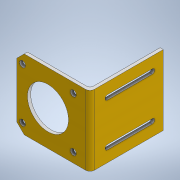
# Autodesk Inventor part: Soporte Motor
Saved by Autodesk Inventor 2021 (Build 250183000, 183)
## iProperties
Created: 2022-01-28
Part Number: Soporte Motor
Material: Generic
Document SubType Name: Modeling
Designer: deuts
Density: 1 g/cm^3
Appearance: Default
Author: deuts
Autodesk Inventor part; units mm, degrees
ref_plane "YZ Plane" through (0, 0, 0) normal (1, 0, 0) x (0, 1, 0)
ref_plane "XZ Plane" through (0, 0, 0) normal (0, 1, 0) x (-1, 0, 0)
ref_plane "XY Plane" through (0, 0, 0) normal (0, 0, 1) x (1, 0, 0)
sketch "Sketch1" plane through (0, 0, 0) normal (0, 1, 0) x (-1, 0, 0)
  line L0 (4, 0) -> (68, 0)
  line L1 (0, -4) -> (0, -68)
  line L2 (68, -3) -> (6, -3)
  line L3 (3, -6) -> (3, -68)
  line L4 (68, 0) -> (68, -3)
  line L5 (3, -68) -> (0, -68)
  arc A0 (4, 0) -> (0, -4) centre (4, -4) ccw
  arc A1 (6, -3) -> (3, -6) centre (6, -6) ccw
  point P0 (0, 0)
  dimension "d0" = 68
  dimension "d1" = 68
  dimension "d2" = 3
  dimension "d3" = 4
  dimension "d4" = 3
  constraints: 12 end point, 4 point on circle, 4 tangent, 2 centre point, 2 point on line, 2 vertical, 1 horizontal, 1 perpendicular, 1 other
  measures "d0" distance of point (0, 0) L0.end
  measures "d1" distance of point (0, 0) L1.end
  measures "d2" distance between parallel lines of L0 L2
  measures "d3" radius of A0
  measures "d4" radius of A1
extrude "Extrusion1" add sketch "Sketch1" along normal blind 65
sketch "Sketch2" plane through (-68, 0, 0) normal (0, 0, 1) x (1, 0, 0)
  circle A0 centre (29, 32.5) radius 19.05
  point P0 (68, 0)
  point P1 (0, 65)
  dimension "d8" = 38.1
  constraints: 1 centre point
  measures "d8" diameter of A0
extrude "Extrusion2" cut sketch "Sketch2" against normal blind 3
sketch "Sketch3" plane through (-68, 0, 0) normal (0, 0, 1) x (1, 0, 0)
  circle A0 centre (5.43, 8.93) radius 2.75
  point P0 (68, 0)
  dimension "d13" = 5.5
  constraints: 1 centre point
  measures "d13" diameter of A0
extrude "Extrusion3" cut sketch "Sketch3" against normal blind 3
pattern_linear "Rectangular Pattern1" count 2 spacing 47.14 along (0, 1, 0) count 2 spacing 47.14 along (1, 0, 0) of "Extrusion3"
sketch "Sketch4" plane through (0, 0, -4) normal (1, 0, 0) x (0, 0, -1)
  arc A0 (53.8, 50.35) -> (53.8, 54.65) centre (53.8, 52.5) ccw
  arc A1 (12.1, 54.65) -> (12.1, 50.35) centre (12.1, 52.5) ccw
  line L0 (53.8, 54.65) -> (12.1, 54.65)
  line L1 (53.8, 50.35) -> (12.1, 50.35)
  line L2 (46.8257, 32.5) -> (19.3775, 32.5)
  arc A2 (53.8, 10.35) -> (53.8, 14.65) centre (53.8, 12.5) ccw
  arc A3 (12.1, 14.65) -> (12.1, 10.35) centre (12.1, 12.5) ccw
  line L3 (53.8, 10.35) -> (12.1, 10.35)
  line L4 (53.8, 14.65) -> (12.1, 14.65)
  point P0 (-4, 0)
  dimension "d24" = 4.3
  dimension "d26" = 4.3
  constraints: 10 end point, 8 point on circle, 6 symmetric about line, 4 centre point, 2 tangent, 1 horizontal, 2 other
  measures "d24" diameter of A0
  measures "d26" diameter of A1
extrude "Extrusion4" cut sketch "Sketch4" against normal blind 3
chamfer "Chamfer1" distance 7 angle 45 2 edges at (-68, 65, -1.5) (-68, 0, -1.5)
body "Solid1"
